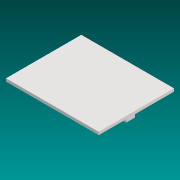
# Autodesk Inventor part: 滑台
Saved by Autodesk Inventor 2021 (Build 250183000, 183)
## iProperties
Created: 2025-04-17
Part Number: 滑台
Material: 常规
Document SubType Name: Modeling
Designer: 86155
Density: 1 g/cm^3
Appearance: 默认
Author: 86155
Autodesk Inventor part; units mm, degrees
ref_plane "YZ Plane" through (0, 0, 0) normal (1, 0, 0) x (0, 1, 0)
ref_plane "XZ Plane" through (0, 0, 0) normal (0, 1, 0) x (-1, 0, 0)
ref_plane "XY Plane" through (0, 0, 0) normal (0, 0, 1) x (1, 0, 0)
sketch "草图1" plane through (0, 0, 0) normal (0, 0, 1) x (1, 0, 0)
  circle A0 centre (0, 0) radius 5
  circle A1 centre (260, 0) radius 5
  line L0 (-10, 15) -> (10, 15)
  line L1 (10, 15) -> (10, -15)
  line L2 (10, -15) -> (-10, -15)
  line L3 (-10, -15) -> (-10, 15)
  line L4 (250, 15) -> (270, 15)
  line L5 (270, 15) -> (270, -15)
  line L6 (270, -15) -> (250, -15)
  line L7 (250, -15) -> (250, 15)
  line L8 (-30, 25) -> (290, 25)
  line L9 (290, 25) -> (290, 15)
  line L10 (290, 15) -> (-30, 15)
  line L11 (-30, 15) -> (-30, 25)
  dimension "d0" = 10
  dimension "d1" = 10
  dimension "d2" = 260
  dimension "d3" = 20
  dimension "d4" = 10
  dimension "d5" = 30
  dimension "d6" = 15
  dimension "d7" = 20
  dimension "d8" = 30
  dimension "d9" = 15
  dimension "d10" = 10
  dimension "d11" = 320
  dimension "d12" = 20
  dimension "d13" = 10
  constraints: 24 end point, 6 parallel, 3 horizontal, 3 perpendicular, 2 centre point, 1 coincident, 1 collinear
  measures "d0" diameter of A0
  measures "d1" diameter of A1
  measures "d2" distance of A1.centre A0.centre
  measures "d3" distance between parallel lines of L1 L3
  measures "d4" distance from line of L1 A0.centre
  measures "d5" distance of L2.end L0.start
  measures "d6" distance from line of L0 A0.centre
  measures "d7" distance of L5.end L6.end
  measures "d8" distance of L4.end L5.end
  measures "d9" distance from line of L4 A1.centre
  measures "d10" distance from line of L7 A1.centre
  measures "d11" distance of L8.start L8.end
  measures "d12" distance between parallel lines of L3 L11
  measures "d13" distance between parallel lines of L10 L8
extrude "拉伸1" add sketch "草图1" along normal blind 30 contours A1 | L0 L1 L2 L3 | L4 L5 L6 L7
extrude "拉伸2" add sketch "草图1" along normal blind 145 and the other way blind 115 contours L10 L11 L8 L9 L4 L0
extrude "拉伸3" cut sketch "草图1" along normal blind 30 contours A1
sketch "草图2" plane through (-30, 15, 145) normal (0, -1, 0) x (1, 0, 0)
  line L0 (309.6956, -155) -> (317.1956, -155)
  line L1 (317.1956, -155) -> (317.1956, -105)
  line L2 (317.1956, -105) -> (309.6956, -105)
  line L3 (309.6956, -105) -> (309.6956, -155)
  line L4 (0, 0) -> (320, 0) projected
  point P0 (30, -145)
  dimension "d22" = 7.5
  dimension "d23" = 105
  dimension "d24" = 50
  constraints: 8 end point, 2 parallel, 1 horizontal, 1 perpendicular
  measures "d22" distance of L2.end L1.end
  measures "d23" distance between parallel lines of L4 L2
  measures "d24" distance between parallel lines of L2 L0
extrude "拉伸4" add sketch "草图2" along normal blind 7
sketch "草图3" plane through (287.1956, 15, 40) normal (1, 0, 0) x (0, 0, -1)
  line L0 (50, 0) -> (50, -7) projected
  line L1 (0, 0) -> (0, -7) projected
  line L2 (50, -7) -> (0, -7)
  line L3 (0, -7) -> (0, -5)
  line L4 (0, -5) -> (50, -5)
  line L5 (50, -5) -> (50, -7)
  point P0 (40, -15)
  dimension "d27" = 2
  constraints: 8 end point, 2 parallel, 1 horizontal, 1 perpendicular, 1 point on line
  measures "d27" distance of L2.end L3.end
extrude "拉伸5" add sketch "草图3" along normal blind 12
